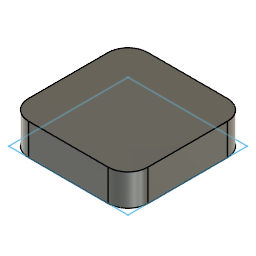
pluviometro (Autodesk Fusion 360 archive; units mm, degrees)
design "sensor aqara"
Autodesk Fusion 360 part; units mm, degrees
note: some values were not read from the file. Set by a fixed rule: which face or edge a step refers to.
sketch "Boceto1" plane through (0, 0, 0) normal (0, 0, 1) x (1, 0, 0)
  line L0 (-16, 16) -> (20, 16)
  line L1 (20, 16) -> (20, -20)
  line L2 (20, -20) -> (-16, -20)
  line L3 (-16, -20) -> (-16, 16)
  dimension "d1" = 36
  constraint horizontal L0
  constraint vertical L1
  constraint horizontal L2
  constraint vertical L3
  constraint equal L0 L3
  measures "d1" distance of L0.start L2.end
extrude "Extruir1" add sketch "Boceto1" along normal blind 9.5
fillet "Empalme1" radius 6 4 edges at (-16, -20, 4.75) (20, -20, 4.75) (20, 16, 4.75) (-16, 16, 4.75)

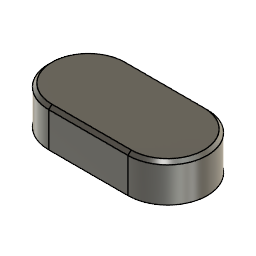
design "sensor"
Autodesk Fusion 360 part; units mm, degrees
sketch "Boceto1" plane through (0, 0, 0) normal (0, 0, 1) x (1, 0, 0)
  line L0 (6.3627, -2.3021) -> (31.3627, -2.3021)
  arc A0 (31.3627, -2.3021) -> (31.3627, 22.6979) centre (31.3627, 10.1979) ccw
  line L1 (31.3627, 22.6979) -> (6.3627, 22.6979)
  arc A1 (6.3627, 22.6979) -> (6.3627, -2.3021) centre (6.3627, 10.1979) ccw
  line L2 (6.3627, 10.1979) -> (31.3627, 10.1979) construction
  point P0 (-6.1373, 10.1979)
  point P1 (43.8627, 10.1979)
  dimension "d1" = 50
  dimension "d2" = 25
  constraint tangent L0 A0
  constraint tangent A0 L1
  constraint parallel L0 L1
  constraint tangent L1 A1
  constraint tangent L0 A1
  constraint horizontal L2
  constraint midpoint A1 P0
  constraint midpoint A0 P1
  measures "d1" distance of P0 P1
  measures "d2" distance of L0 L1
extrude "Extruir1" add sketch "Boceto1" along normal blind 12
chamfer "Chaflán1" distance 1 angle 45 4 edges at (-6.1373, 10.1979, 12) (18.8627, -2.3021, 12) (43.8627, 10.1979, 12) (18.8627, 22.6979, 12)

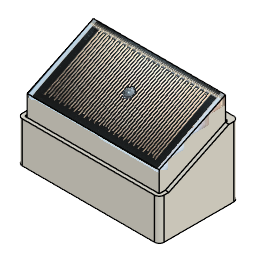
design "pluviometro"
Autodesk Fusion 360 part; units mm, degrees
sketch "Boceto1" plane through (0, 0, 0) normal (0, 0, 1) x (1, 0, 0)
  line L0 (-27.5, 16.5) -> (27.5, 16.5)
  line L1 (29.5, 14.5) -> (29.5, -14.5)
  line L2 (27.5, -16.5) -> (-27.5, -16.5)
  line L3 (-29.5, -14.5) -> (-29.5, 14.5)
  line L4 (-29.5, 0) -> (29.5, 0) construction
  arc A0 (-27.5, 16.5) -> (-29.5, 14.5) centre (-27.5, 14.5) ccw
  arc A1 (29.5, 14.5) -> (27.5, 16.5) centre (27.5, 14.5) ccw
  arc A2 (-29.5, -14.5) -> (-27.5, -16.5) centre (-27.5, -14.5) ccw
  arc A3 (27.5, -16.5) -> (29.5, -14.5) centre (27.5, -14.5) ccw
  dimension "d1" = 59
  dimension "d2" = 33
  dimension "d3" = 2
  constraint horizontal L0
  constraint vertical L1
  constraint horizontal L2
  constraint vertical L3
  constraint midpoint origin L4
  constraint coincident L3 L4.start
  constraint tangent L0 A0
  constraint tangent L3 A0
  constraint coincident L1 L4.end
  constraint tangent L0 A1
  constraint tangent L1 A1
  constraint equal A0 A1
  constraint tangent L3 A2
  constraint tangent L2 A2
  constraint equal A0 A2
  constraint tangent L2 A3
  constraint tangent L1 A3
  constraint equal A0 A3
  constraint midpoint L3 L4.start
  constraint horizontal L4
  measures "d1" distance of L1 L3
  measures "d2" distance of L0 L2
  measures "d3" radius of A0
extrude "Extruir1" add sketch "Boceto1" along normal blind 30
sketch "Boceto2" plane through (0, 0, 0) normal (1, 0, 0) x (0, 1, 0)
  line L0 (16.5, 29) -> (12.5, 29)
  line L1 (12.5, 29) -> (-12.5, 17)
  line L2 (-12.5, 17) -> (-16.5, 17)
  line L3 (-16.5, 30) -> (16.5, 30)
  line L4 (16.5, 29) -> (16.5, 30)
  line L5 (-16.5, 17) -> (-16.5, 30)
  line L6 (16.5, 62.061) -> (16.5, 40)
  line L7 (16.5, 40) -> (-16.5, 24.16)
  line L8 (-16.5, 24.16) -> (-16.5, 62.061)
  line L9 (-16.5, 62.061) -> (16.5, 62.061)
  point P0 (16.5, 30)
  point P1 (-16.5, 0)
  point P2 (-16.5, 0)
  dimension "d6" = 1
  dimension "d7" = 4
  dimension "d8" = 17
  dimension "d16" = 40
  constraint horizontal L0
  constraint vertical L4
  constraint coincident P0 L3.end
  constraint equal L0 L2
  constraint horizontal L3
  constraint vertical L5
  constraint coincident P2 L5
  constraint horizontal L2
  constraint vertical L6
  constraint parallel L6 L8
  constraint horizontal L9
  constraint parallel L1 L7
  constraint coincident L0.start L6
  constraint coincident L5 L7.end
  measures "d6" distance of L0.start P0
  measures "d7" distance of L0.start L0.end
  measures "d8" distance of L2 P2
  measures "d16" vertical distance of L6.end P2
shell "Vaciado1" thickness 1.5 removed faces 1 at (9.1667, -5.5, 30)
move_face "CarasDesfase1" offset 1.4 1 faces at (-9.1667, 15, 20.5)
extrude "Extruir2" cut sketch "Boceto2" along normal through all and the other way through all contours L0 L1 L2 L3 L4 L5 L7 | L3 L5 L7 L8
sketch "Boceto4" plane through (0, 0, 1.5) normal (0, 0, 1) x (-1, 0, 0)
  arc A0 (27.5, -13.6) -> (28, -13.1) centre (27.5, -13.1) ccw
  line L0 (28, -13.1) -> (28, 14.5)
  arc A1 (28, 14.5) -> (27.5, 15) centre (27.5, 14.5) ccw
  line L1 (27.5, 15) -> (-27.5, 15)
  arc A2 (-27.5, 15) -> (-28, 14.5) centre (-27.5, 14.5) ccw
  line L2 (-28, 14.5) -> (-28, -13.1)
  arc A3 (-28, -13.1) -> (-27.5, -13.6) centre (-27.5, -13.1) ccw
  line L3 (-27.5, -13.6) -> (27.5, -13.6)
  line L4 (27.5, 14.5) -> (-27.5, 14.5)
  line L5 (-27.5, 14.5) -> (-27.5, -13.1)
  line L6 (-27.5, -13.1) -> (27.5, -13.1)
  line L7 (27.5, -13.1) -> (27.5, 14.5)
  line L8 (0, 14.5) -> (0, -13.1) construction
  circle A4 centre (0, 1) radius 1.5
  dimension "d12" = -0.5
  dimension "d18" = 3
  dimension "d19" = 1
  constraint midpoint L4 L8.start
  constraint midpoint L6 L8.end
  constraint coincident L8 A4.centre
  measures "d18" diameter of A4
  measures "d19" distance of origin A4.centre
extrude "Extruir5" cut sketch "Boceto4" against normal through all contours A4
extrude "Extruir3" add sketch "Boceto4" along normal blind 40 contours L4 L5 L6 L7 | A4
extrude "Extruir4" cut sketch "Boceto2" along normal through all and the other way through all contours L3 L5 L7 L8 | L3 L6 L7 L8 L9
